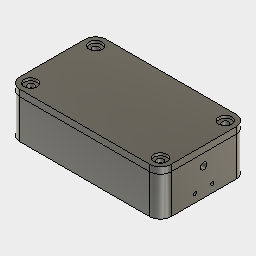
BoxAladinMouse (Autodesk Fusion 360 design; units mm, degrees)
Autodesk Fusion 360 part; units mm, degrees
note: some values were not read from the file. Set by a fixed rule: which sketch regions a step uses.
sketch "Sketch1" plane through (0, 0, 0) normal (0, 0, 1) x (1, 0, 0)
  line L0 (0, 0) -> (70, 0)
  line L1 (70, 0) -> (70, 40)
  line L2 (70, 40) -> (0, 40)
  line L3 (0, 40) -> (0, 0)
  dimension "d1" = 40
  dimension "d2" = 70
  measures "d1" distance of L0.start L2.end
  measures "d2" distance of L0.start L0.end
extrude "Extrude1" add sketch "Sketch1" against normal blind 3 makes body 1
sketch "Sketch2" plane through (0, 0, 0) normal (0, 0, 1) x (-1, 0, 0)
  line L0 (0, -40) -> (0, 0)
  line L1 (0, 0) -> (-70, 0)
  line L2 (-70, 0) -> (-70, -40)
  line L3 (-70, -40) -> (0, -40)
  line L4 (-67, -37) -> (-3, -37)
  line L5 (-3, -37) -> (-3, -3)
  line L6 (-3, -3) -> (-67, -3)
  line L7 (-67, -3) -> (-67, -37)
  dimension "d5" = 3
extrude "Extrude2" add sketch "Sketch2" along normal blind 15 bodies 1
sketch "Sketch3" plane through (0, 0, 0) normal (-1, 0, 0) x (0, -1, 0)
  line L0 (-40, 15) -> (-40, -3)
  line L1 (-40, -3) -> (0, -3)
  line L2 (0, -3) -> (0, 15)
  line L3 (0, 15) -> (-40, 15)
  line L4 (-24, 6) -> (-16, 6)
  line L5 (-16, 6) -> (-16, 3)
  line L6 (-16, 3) -> (-24, 3)
  line L7 (-24, 3) -> (-24, 6)
  line L8 (-37, 0) -> (-3, 0)
  point P0 (-20, 0)
  point P1 (-20, 3)
  dimension "d8" = 8
  dimension "d9" = 3
  dimension "d10" = 3
  dimension "d11" = 9.5
  measures "d8" distance of L4.start L4.end
  measures "d9" distance of L4.start L6.end
  measures "d10" distance of L6 L8
extrude "Extrude3" cut sketch "Sketch3" against normal up to surface (3 mm away) contours L4 L5 L6 L7 bodies 1
sketch "Sketch4" plane through (3, 0, 0) normal (1, 0, 0) x (0, 1, 0)
  line L0 (24, 6) -> (24, 3)
  line L1 (24, 3) -> (16, 3)
  line L2 (16, 3) -> (16, 6)
  line L3 (16, 6) -> (24, 6)
  line L4 (3, 0) -> (37, 0)
  line L5 (37, 0) -> (37, 15)
  line L6 (37, 15) -> (3, 15)
  line L7 (3, 15) -> (3, 0)
  line L8 (3, 7.5) -> (37, 7.5)
  line L9 (37, 7.5) -> (37, 0)
  line L10 (37, 0) -> (3, 0)
  line L11 (3, 0) -> (3, 7.5)
extrude "Extrude4" cut sketch "Sketch4" against normal blind 1 contours L4 L5 L7 L8 L9 L10 L11 bodies 1
chamfer "Chamfer1" distance 1 angle 45 1 edges at (3, 20, 7.5) on bodies 1
sketch "Sketch5" plane through (0, 0, 0) normal (0, 0, 1) x (-1, 0, 0)
  line L0 (-67, -37) -> (-2, -37)
  line L1 (-2, -37) -> (-2, -3)
  line L2 (-2, -3) -> (-67, -3)
  line L3 (-67, -3) -> (-67, -37)
  line L4 (-67, -37) -> (-47, -37)
  line L5 (-47, -37) -> (-47, -29)
  line L6 (-47, -29) -> (-67, -29)
  line L7 (-67, -29) -> (-67, -37)
  line L8 (-2, -37) -> (-14, -37)
  line L9 (-14, -37) -> (-14, -29)
  line L10 (-14, -29) -> (-2, -29)
  line L11 (-2, -29) -> (-2, -37)
  line L12 (-67, -20) -> (-2, -20) construction
  line L13 (-2, -3) -> (-14, -3)
  line L14 (-14, -3) -> (-14, -11)
  line L15 (-14, -11) -> (-2, -11)
  line L16 (-2, -11) -> (-2, -3)
  line L17 (-67, -3) -> (-47, -3)
  line L18 (-47, -3) -> (-47, -11)
  line L19 (-67, -11) -> (-67, -3)
  line L20 (-47, -11) -> (-67, -11)
  dimension "d17" = 9
  dimension "d18" = 20
  dimension "d19" = 12
  measures "d17" distance of L6 L12
  measures "d18" distance of L5.end L6.end
  measures "d19" distance of L9.end L10.end
extrude "Extrude5" add sketch "Sketch5" along normal up to surface (2 mm away) contours L0 L3 L4 L5 L6 L7 | L0 L1 L8 L9 L10 L11 | L2 L3 L17 L18 L19 L20 | L1 L2 L13 L14 L15 L16 bodies 1
sketch "Sketch6" plane through (0, 0, 2) normal (0, 0, 1) x (-1, 0, 0)
  line L0 (-47, -29) -> (-67, -29)
  line L1 (-67, -29) -> (-67, -37)
  line L2 (-67, -37) -> (-47, -37)
  line L3 (-47, -37) -> (-47, -29)
  line L4 (-55, -29) -> (-55, -31.75)
  line L5 (-55, -31.75) -> (-47, -31.75)
  line L6 (-67, -11) -> (-67, -29)
  line L7 (-3, -3) -> (-3, -37)
  line L8 (-67, -20) -> (-3, -20) construction
  line L9 (-2, -3) -> (-2, -37)
  line L10 (-55, -11) -> (-55, -8.25)
  line L11 (-55, -8.25) -> (-47, -8.25)
  circle A0 centre (-55, -31.75) radius 1
  circle A1 centre (-55, -8.25) radius 1
  line L12 (-67, -11) -> (-47, -11)
  line L13 (-47, -11) -> (-47, -3)
  line L14 (-47, -3) -> (-67, -3)
  line L15 (-67, -3) -> (-67, -11)
  dimension "d22" = 11.75
  dimension "d23" = 53
  dimension "d24" = 2
  measures "d22" distance of L5 L8
  measures "d23" distance of L4 L9
  measures "d24" diameter of A0
extrude "Extrude6" add sketch "Sketch6" along normal blind 2 contours L0 L1 L2 L3 L4 L5 A0 | L10 L11 A1 L12 L13 L14 L15 bodies 1
fillet "Fillet1" radius 5 10 edges at (0, 0, 6) (70, 0, 6) (70, 40, 6) (0, 40, 6) (67, 3, 9.5) (67, 37, 9.5) (3, 37, 11.75) (2, 37, 4.75) (3, 3, 11.75) (2, 3, 4.75) on bodies 1
sketch "Sketch7" plane through (0, 0, 15) normal (0, 0, 1) x (-1, 0, 0)
  line L0 (-67, -32) -> (-67, -8)
  arc A0 (-62, -3) -> (-67, -8) centre (-62, -8) ccw
  line L1 (-62, -3) -> (-8, -3)
  arc A1 (-3, -8) -> (-8, -3) centre (-8, -8) ccw
  line L2 (-3, -8) -> (-3, -32)
  arc A2 (-8, -37) -> (-3, -32) centre (-8, -32) ccw
  line L3 (-8, -37) -> (-62, -37)
  arc A3 (-67, -32) -> (-62, -37) centre (-62, -32) ccw
  arc A4 (-5, -40) -> (0, -35) centre (-5, -35) ccw
  line L4 (0, -35) -> (0, -5)
  arc A5 (0, -5) -> (-5, 0) centre (-5, -5) ccw
  line L5 (-5, 0) -> (-65, 0)
  arc A6 (-65, 0) -> (-70, -5) centre (-65, -5) ccw
  line L6 (-70, -5) -> (-70, -35)
  arc A7 (-70, -35) -> (-65, -40) centre (-65, -35) ccw
  line L7 (-65, -40) -> (-5, -40)
  line L8 (-67, -32.5) -> (-60, -32.5)
  line L9 (-60, -32.5) -> (-60, -37)
  line L10 (-3, -32.5) -> (-9, -32.5)
  line L11 (-9, -32.5) -> (-9, -37)
  line L12 (-67, -20) -> (-3, -20) construction
  line L13 (-67, -7.5) -> (-60, -7.5)
  line L14 (-60, -7.5) -> (-60, -3)
  line L15 (-3, -7.5) -> (-9, -7.5)
  line L16 (-9, -7.5) -> (-9, -3)
  arc A8 (-7, -37) -> (-2, -32) centre (-7, -32) ccw
  line L17 (-3, -32.5) -> (-2.0251, -32.5)
  line L18 (-3, -7.5) -> (-2.0251, -7.5)
  line L19 (-7, -37) -> (-9, -37)
  arc A9 (-2, -8) -> (-7, -3) centre (-7, -8) ccw
  line L20 (-7, -3) -> (-9, -3)
  dimension "d28" = 12.5
  dimension "d30" = 6
  dimension "d31" = 7
  measures "d28" distance of L8 L12
  measures "d30" distance of L10.start L10.end
  measures "d31" distance of L8.start L8.end
extrude "Extrude7" add sketch "Sketch7" against normal blind 15 contours L3 A3 L8 L9 | A0 L1 L13 L14 | A2 L3 L10 L11 L19 | L1 A1 L15 L16 L20 | A2 L10 A8 L17 L19 | A1 L15 L18 A9 L20 bodies 1
fillet "Fillet2" radius 3 4 edges at (9, 32.5, 8.5) (9, 7.5, 8.5) (60, 7.5, 9.5) (60, 32.5, 9.5) on bodies 1
fillet "Fillet3" radius 2 4 edges at (14, 29, 1) (47, 29, 1) (47, 11, 1) (14, 11, 1) on bodies 1
sketch "Sketch8" plane through (0, 0, 15) normal (0, 0, 1) x (-1, 0, 0)
  arc A0 (-60, -35.5) -> (-63, -32.5) centre (-63, -35.5) ccw
  line L0 (-63, -32.5) -> (-66.9749, -32.5)
  arc A1 (-67, -32) -> (-66.9749, -32.5) centre (-62, -32) ccw
  line L1 (-67, -32) -> (-67, -8)
  arc A2 (-66.9749, -7.5) -> (-67, -8) centre (-62, -8) ccw
  line L2 (-66.9749, -7.5) -> (-63, -7.5)
  arc A3 (-63, -7.5) -> (-60, -4.5) centre (-63, -4.5) ccw
  line L3 (-60, -4.5) -> (-60, -3)
  line L4 (-60, -3) -> (-9, -3)
  line L5 (-9, -3) -> (-9, -4.5)
  arc A4 (-9, -4.5) -> (-6, -7.5) centre (-6, -4.5) ccw
  line L6 (-6, -7.5) -> (-3.0251, -7.5)
  arc A5 (-3, -8) -> (-3.0251, -7.5) centre (-8, -8) ccw
  line L7 (-3, -8) -> (-3, -32)
  arc A6 (-3.0251, -32.5) -> (-3, -32) centre (-8, -32) ccw
  line L8 (-3.0251, -32.5) -> (-6, -32.5)
  arc A7 (-6, -32.5) -> (-9, -35.5) centre (-6, -35.5) ccw
  line L9 (-9, -35.5) -> (-9, -37)
  line L10 (-9, -37) -> (-60, -37)
  line L11 (-60, -37) -> (-60, -35.5)
  arc A8 (-5, -40) -> (0, -35) centre (-5, -35) ccw
  line L12 (0, -35) -> (0, -5)
  arc A9 (0, -5) -> (-5, 0) centre (-5, -5) ccw
  line L13 (-5, 0) -> (-65, 0)
  arc A10 (-65, 0) -> (-70, -5) centre (-65, -5) ccw
  line L14 (-70, -5) -> (-70, -35)
  arc A11 (-70, -35) -> (-65, -40) centre (-65, -35) ccw
  line L15 (-65, -40) -> (-5, -40)
  circle A12 centre (-5, -35) radius 3 construction
  circle A13 centre (-65, -35) radius 3 construction
  line L16 (-67, -20) -> (-3, -20) construction
  circle A14 centre (-5, -5) radius 3 construction
  circle A15 centre (-65, -5) radius 3 construction
  circle A16 centre (-5, -35) radius 1
  circle A17 centre (-65, -35) radius 1
  circle A18 centre (-65, -5) radius 1
  circle A19 centre (-5, -5) radius 1
  dimension "d36" = 6
  dimension "d37" = 6
  dimension "d38" = 2
  measures "d36" diameter of A12
  measures "d37" diameter of A13
  measures "d38" diameter of A16
extrude "Extrude8" cut sketch "Sketch8" against normal blind 9 contours A16 | A17 | A18 | A19 bodies 1
sketch "Sketch9" plane through (70, 0, 0) normal (1, 0, 0) x (0, 1, 0)
  line L0 (35, -3) -> (35, 15)
  line L1 (35, 15) -> (5, 15)
  line L2 (5, 15) -> (5, -3)
  line L3 (5, -3) -> (35, -3)
  circle A0 centre (16, 0.75) radius 0.75
  line L4 (40, 15) -> (40, -3)
  line L5 (40, -3) -> (40, 15)
  line L6 (0, 0) -> (40, 0) construction
  line L7 (20, 0) -> (20, 2) construction
  circle A1 centre (24, 0.75) radius 0.75
  point P0 (20, 0)
  dimension "d41" = 1.5
  dimension "d42" = 4
  measures "d41" diameter of A0
  measures "d42" distance of A0.centre P0
extrude "Extrude9" cut sketch "Sketch9" against normal blind 4 contours A0 | A1 bodies 1
sketch "Sketch10" plane through (0, 0, 0) normal (0, 0, 1) x (-1, 0, 0)
  line L0 (-67, -29) -> (-49, -29)
  arc A0 (-47, -31) -> (-49, -29) centre (-49, -31) ccw
  line L1 (-47, -31) -> (-47, -37)
  line L2 (-47, -37) -> (-14, -37)
  line L3 (-14, -37) -> (-14, -31)
  arc A1 (-12, -29) -> (-14, -31) centre (-12, -31) ccw
  line L4 (-12, -29) -> (-2, -29)
  line L5 (-2, -29) -> (-2, -11)
  line L6 (-2, -11) -> (-12, -11)
  arc A2 (-14, -9) -> (-12, -11) centre (-12, -9) ccw
  line L7 (-14, -9) -> (-14, -3)
  line L8 (-14, -3) -> (-47, -3)
  line L9 (-47, -3) -> (-47, -9)
  arc A3 (-49, -11) -> (-47, -9) centre (-49, -9) ccw
  line L10 (-49, -11) -> (-67, -11)
  line L11 (-67, -11) -> (-67, -16)
  line L12 (-67, -16) -> (-67, -24)
  line L13 (-67, -24) -> (-67, -29)
  line L14 (-67, -24) -> (-55, -24) construction
  line L15 (-67, -16) -> (-55, -16) construction
  circle A4 centre (-61, -25.7) radius 2
  line L16 (-63.5467, -27.7) -> (-58.5467, -27.7) construction
  line L17 (-67, -20) -> (-55, -20) construction
  circle A5 centre (-61, -14.3) radius 2
  dimension "d45" = 4
  dimension "d46" = 1.3
  dimension "d47" = 6
  measures "d45" diameter of A4
  measures "d46" distance of L0 L16
  measures "d47" distance of L13 A4.centre
extrude "Extrude10" add sketch "Sketch10" along normal blind 4 contours A4 | A5 bodies 1
fillet "Fillet4" radius 0.8 4 edges at (1, 16, 6) (1, 24, 6) (1, 24, 3) (1, 16, 3) on bodies 1
sketch "Sketch11" plane through (0, 0, 15) normal (0, 0, 1) x (-1, 0, 0)
  circle A0 centre (-5, -5) radius 1
  circle A1 centre (-65, -5) radius 1
  circle A2 centre (-5, -35) radius 1
  circle A3 centre (-65, -35) radius 1
  arc A4 (-60, -35.5) -> (-63, -32.5) centre (-63, -35.5) ccw
  line L0 (-63, -32.5) -> (-66.9749, -32.5)
  arc A5 (-67, -32) -> (-66.9749, -32.5) centre (-62, -32) ccw
  line L1 (-67, -32) -> (-67, -8)
  arc A6 (-66.9749, -7.5) -> (-67, -8) centre (-62, -8) ccw
  line L2 (-66.9749, -7.5) -> (-63, -7.5)
  arc A7 (-63, -7.5) -> (-60, -4.5) centre (-63, -4.5) ccw
  line L3 (-60, -4.5) -> (-60, -3)
  line L4 (-60, -3) -> (-9, -3)
  line L5 (-9, -3) -> (-9, -4.5)
  arc A8 (-9, -4.5) -> (-6, -7.5) centre (-6, -4.5) ccw
  line L6 (-6, -7.5) -> (-3.0251, -7.5)
  arc A9 (-3, -8) -> (-3.0251, -7.5) centre (-8, -8) ccw
  line L7 (-3, -8) -> (-3, -32)
  arc A10 (-3.0251, -32.5) -> (-3, -32) centre (-8, -32) ccw
  line L8 (-3.0251, -32.5) -> (-6, -32.5)
  arc A11 (-6, -32.5) -> (-9, -35.5) centre (-6, -35.5) ccw
  line L9 (-9, -35.5) -> (-9, -37)
  line L10 (-9, -37) -> (-60, -37)
  line L11 (-60, -37) -> (-60, -35.5)
  arc A12 (-5, -40) -> (0, -35) centre (-5, -35) ccw
  line L12 (0, -35) -> (0, -5)
  arc A13 (0, -5) -> (-5, 0) centre (-5, -5) ccw
  line L13 (-5, 0) -> (-65, 0)
  arc A14 (-65, 0) -> (-70, -5) centre (-65, -5) ccw
  line L14 (-70, -5) -> (-70, -35)
  arc A15 (-70, -35) -> (-65, -40) centre (-65, -35) ccw
  line L15 (-65, -40) -> (-5, -40)
  circle A16 centre (-5, -35) radius 1.5
  circle A17 centre (-65, -35) radius 1.5
  circle A18 centre (-65, -5) radius 1.5
  circle A19 centre (-5, -5) radius 1.5
  dimension "d56" = 3
  measures "d56" diameter of A16
extrude "Extrude11" add sketch "Sketch11" along normal blind 3 separate body contours A4 L0 A5 L1 A6 L2 A7 L3 L4 L5 A8 L6 A9 L7 A10 L8 A11 L9 L10 L11 | A12 L12 A13 L13 A14 L14 A15 L15 makes body 2
sketch "Sketch12" plane through (0, 0, 18) normal (0, 0, 1) x (-1, 0, 0)
  line L0 (-65, -40) -> (-5, -40)
  arc A0 (-5, -40) -> (0, -35) centre (-5, -35) ccw
  line L1 (0, -35) -> (0, -5)
  arc A1 (0, -5) -> (-5, 0) centre (-5, -5) ccw
  line L2 (-5, 0) -> (-65, 0)
  arc A2 (-65, 0) -> (-70, -5) centre (-65, -5) ccw
  line L3 (-70, -5) -> (-70, -35)
  arc A3 (-70, -35) -> (-65, -40) centre (-65, -35) ccw
  circle A4 centre (-5, -35) radius 3
  circle A5 centre (-65, -35) radius 3
  circle A6 centre (-65, -5) radius 3
  circle A7 centre (-5, -5) radius 3
  circle A8 centre (-65, -35) radius 1.5
  circle A9 centre (-5, -5) radius 1.5
  circle A10 centre (-5, -35) radius 1.5
  circle A11 centre (-65, -5) radius 1.5
  dimension "d53" = 6
  measures "d53" diameter of A4
extrude "Extrude12" cut sketch "Sketch12" against normal blind 1.2 contours A4 | A5 | A6 | A7 bodies 2
sketch "Sketch13" plane through (70, 0, 0) normal (1, 0, 0) x (0, 1, 0)
  circle A0 centre (24, 0.75) radius 0.75
  circle A1 centre (16, 0.75) radius 0.75
  line L0 (35, -3) -> (35, 15)
  line L1 (35, 15) -> (5, 15)
  line L2 (5, 15) -> (5, -3)
  line L3 (5, -3) -> (35, -3)
  circle A2 centre (20, 9.7793) radius 1.5
  dimension "d57" = 3
  measures "d57" diameter of A2
extrude "Extrude13" cut sketch "Sketch13" against normal up to surface (3 mm away) contours A2 bodies 1
equation "d17 = ( 18 / 2 ) * 1 mm"
equation "d22 = ( 23.5 / 2 ) * 1 mm"
equation "d28 = ( 23 / 2 ) * 1 mm + 1 mm"
